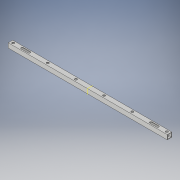
# Autodesk Inventor part: holder_bar
Saved by Autodesk Inventor 2019 (Build 230136000, 136)
## iProperties
Created: 2019-02-02
Part Number: holder_bar
Material: Generic
Document SubType Name: Modeling
Designer: suchanek
Density: 1 g/cm^3
Appearance: Default
Author: suchanek
Autodesk Inventor part; units mm, degrees
ref_plane "XZ Plane" through (0, 0, 0) normal (0, 1, 0) x (-1, 0, 0)
ref_plane "XY Plane" through (0, 0, 0) normal (0, 0, 1) x (1, 0, 0)
sketch "Sketch1" plane through (0, 0, 0) normal (1, 0, 0) x (0, 1, 0)
  line L0 (-5, 5) -> (5, 5)
  line L1 (5, 5) -> (5, -5)
  line L2 (5, -5) -> (-5, -5)
  line L3 (-5, -5) -> (-5, 5)
  line L4 (-5, 5) -> (5, -5) construction
  line L5 (5, 5) -> (-5, -5) construction
  line L6 (-4, 4) -> (4, 4)
  line L7 (4, 4) -> (4, -4)
  line L8 (4, -4) -> (-4, -4)
  line L9 (-4, -4) -> (-4, 4)
  line L10 (-4, 4) -> (4, -4) construction
  line L11 (4, 4) -> (-4, -4) construction
  point P0 (0, 0)
  dimension "d0" = 10
  dimension "d1" = 10
  dimension "d2" = 8
  dimension "d3" = 8
  constraints: 24 end point, 4 midpoint, 4 parallel, 2 horizontal, 2 perpendicular
  measures "d0" distance of L1.end L2.end
  measures "d1" distance of L0.end L1.end
  measures "d2" distance of L7.end L8.end
  measures "d3" distance of L6.end L7.end
extrude "Extrusion1" add sketch "Sketch1" along normal mid plane 350
sketch "Sketch2" plane through (-175, 5, 5) normal (0, 1, 0) x (1, 0, 0)
  circle A0 centre (6, 5) radius 2.6
  line L0 (26, 5) -> (41, 5) construction
  line L1 (26, 2.4) -> (41, 2.4)
  line L2 (41, 7.6) -> (26, 7.6)
  arc A1 (26, 7.6) -> (26, 2.4) centre (26, 5) ccw
  arc A2 (41, 2.4) -> (41, 7.6) centre (41, 5) ccw
  line L3 (0, 0) -> (0, 10) projected
  circle A3 centre (82, 5) radius 2.6
  circle A4 centre (144, 5) radius 2.6
  point P0 (175, 5)
  point P1 (33.5, 5)
  dimension "d6" = 5.2
  dimension "d7" = 6
  dimension "d8" = 20
  dimension "d9" = 15
  dimension "d13" = 62
  dimension "d14" = 31
  constraints: 8 end point, 5 centre point, 4 point on circle, 4 point on line, 4 tangent, 3 equal radius, 1 horizontal, 1 midpoint, 1 parallel
  measures "d6" diameter of A0
  measures "d7" distance from line of L3 A0.centre
  measures "d8" distance of A0.centre L0.start
  measures "d9" distance of L2.start L2.end
  measures "d13" distance of A3.centre A4.centre
  measures "d14" distance of point (175, 5) A4.centre
extrude "Extrusion2" cut sketch "Sketch2" against normal blind 100
mirror "Mirror1" about plane through (0, 0, 0) normal (1, 0, 0) of "Extrusion2"
body "Solid1"
